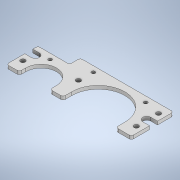
# Autodesk Inventor part: Bottle clamping plate 1
Saved by Autodesk Inventor 2021 (Build 250183000, 183)
## iProperties
Created: 2020-07-28
Part Number: Bottle clamping plate 1
Material: Generic
Document SubType Name: Modeling
Designer: jgray
Density: 1 g/cm^3
Appearance: Default
Author: jgray
Autodesk Inventor part; units mm, degrees
ref_plane "YZ Plane" through (0, 0, 0) normal (1, 0, 0) x (0, 1, 0)
ref_plane "XZ Plane" through (0, 0, 0) normal (0, 1, 0) x (-1, 0, 0)
ref_plane "XY Plane" through (0, 0, 0) normal (0, 0, 1) x (1, 0, 0)
sketch "Sketch1" plane through (0, 0, 0) normal (0, 1, 0) x (-1, 0, 0)
  line L0 (-56.25, 58.25) -> (56.25, 58.25)
  line L1 (56.25, 58.25) -> (56.25, -58.25)
  line L2 (56.25, -58.25) -> (-56.25, -58.25)
  line L3 (-56.25, -58.25) -> (-56.25, 58.25)
  line L4 (-56.25, 58.25) -> (56.25, -58.25) construction
  line L5 (56.25, 58.25) -> (-56.25, -58.25) construction
  point P0 (0, 0)
  dimension "d0" = 112.5
  dimension "d1" = 116.5
  constraints: 12 end point, 2 midpoint, 2 parallel, 1 horizontal, 1 perpendicular
  measures "d0" distance of L1.end L2.end
  measures "d1" distance of L0.end L1.end
extrude "Extrusion1" add sketch "Sketch1" along normal blind 3
sketch "Sketch2" plane through (0, 3, 0) normal (0, 1, 0) x (1, 0, 0)
  circle A0 centre (18.5, 28) radius 23.85
  circle A1 centre (37, -23.25) radius 13.85
  circle A2 centre (-35, -40.25) radius 13.85
  circle A3 centre (-30.9, 25.8) radius 13.85
  circle A4 centre (0, -23.25) radius 13.85
  line L0 (56.25, 58.25) -> (-56.25, 58.25) projected
  line L1 (-56.25, -58.25) -> (56.25, -58.25) projected
  line L2 (0, -105.9299) -> (0, 123.2086) construction
  line L3 (-76.4777, -40.25) -> (-5.35, -40.25) construction
  line L4 (-123.5447, -23.25) -> (82.5572, -23.25) construction
  line L5 (56.25, -58.25) -> (56.25, 58.25) construction
  point P0 (0, 0)
  dimension "d4" = 47.7
  dimension "d5" = 27.7
  dimension "d6" = 27.7
  dimension "d7" = 27.7
  dimension "d8" = 27.7
  dimension "d9" = 116.5
  dimension "d10" = 112.5
  dimension "d13" = 37
  dimension "d14" = 18.5
  dimension "d15" = 30.9
  dimension "d18" = 18
  dimension "d19" = 35
  dimension "d20" = 35
  dimension "d53" = 28
  dimension "d54" = 25.8
  constraints: 6 end point, 5 centre point, 5 point on line, 1 horizontal, 1 perpendicular, 1 vertical
  measures "d4" diameter of A0
  measures "d5" diameter of A1
  measures "d6" diameter of A2
  measures "d7" diameter of A3
  measures "d8" diameter of A4
  measures "d9" distance between parallel lines of L0 L1
  measures "d10" distance of L1.start L1.end
  measures "d13" distance of A4.centre A1.centre
  measures "d14" distance from line of A0.centre L2
  measures "d15" distance from line of A3.centre L2
  measures "d18" distance between parallel lines of L1 L3
  measures "d19" distance between parallel lines of L1 L4
  measures "d20" horizontal distance of A2.centre A4.centre
  measures "d53" vertical distance of point (0, 0) A0.centre
  measures "d54" vertical distance of point (0, 0) A3.centre
extrude "Extrusion2" cut sketch "Sketch2" against normal blind 5
sketch "Sketch4" plane through (0, 3, 0) normal (0, 1, 0) x (1, 0, 0)
  line L0 (-56.25, 58.25) -> (-56.25, -58.25)
  line L1 (56.25, -58.25) -> (56.25, 58.25)
  line L2 (18.5, -17.4904) -> (18.5, -40.0394) construction
  line L3 (-51.55, 5.4) -> (-51.55, 71.9941) construction
  line L4 (50.75, 5.4) -> (50.75, 69.4565) construction
  line L5 (-73.722, 50) -> (66.5467, 50) construction
  line L6 (66.5467, 30) -> (-76.0779, 30) construction
  circle A0 centre (18.5, 28) radius 23.85
  circle A1 centre (37, -23.25) radius 13.85
  circle A2 centre (-30.9, 25.8) radius 13.85
  circle A3 centre (0, -23.25) radius 13.85
  circle A4 centre (-35, -40.25) radius 13.85
  line L7 (56.25, 58.25) -> (-56.25, 58.25)
  line L8 (-56.25, 58.25) -> (-56.25, -58.25)
  line L9 (-56.25, -58.25) -> (56.25, -58.25)
  line L10 (56.25, -58.25) -> (56.25, 58.25)
  circle A5 centre (-30.9, 25.8) radius 13.85
  circle A6 centre (18.5, 28) radius 23.85
  circle A7 centre (0, -23.25) radius 13.85
  circle A8 centre (37, -23.25) radius 13.85
  circle A9 centre (-35, -40.25) radius 13.85
  line L11 (-56.25, 58.25) -> (-56.25, -58.25)
  line L12 (-56.25, 58.25) -> (-56.25, -58.25)
  line L13 (56.25, -58.25) -> (56.25, 58.25)
  line L14 (56.25, 58.25) -> (56.25, -58.25)
  line L15 (-56.25, 20) -> (-44.75, 20)
  line L16 (-17.05, 20) -> (-5.35, 20)
  line L17 (42.35, 20) -> (56.25, 20)
  line L18 (-56.25, -40.25) -> (-48.85, -40.25)
  circle A10 centre (-35, -40.25) radius 13.85
  circle A11 centre (37, -23.25) radius 13.85
  line L19 (50.85, -23.25) -> (56.25, -23.25)
  circle A12 centre (0, -23.25) radius 13.85
  line L20 (-13.85, -23.25) -> (-13.85, -38.25)
  line L21 (-15.85, -40.25) -> (-21.15, -40.25)
  line L22 (13.85, -23.25) -> (13.85, -31.25)
  line L23 (15.85, -33.25) -> (21.15, -33.25)
  line L24 (23.15, -31.25) -> (23.15, -23.25)
  arc A13 (13.85, -31.25) -> (15.85, -33.25) centre (15.85, -31.25) ccw
  arc A14 (21.15, -33.25) -> (23.15, -31.25) centre (21.15, -31.25) ccw
  arc A15 (-15.85, -40.25) -> (-13.85, -38.25) centre (-15.85, -38.25) ccw
  line L25 (-44.75, 25.8) -> (-44.75, 20)
  circle A16 centre (-30.9, 25.8) radius 13.85 projected
  line L26 (-17.05, 25.8) -> (-17.05, 20)
  line L27 (-5.35, 28) -> (-5.35, 20)
  circle A17 centre (18.5, 28) radius 23.85 projected
  line L28 (42.35, 28) -> (42.35, 20)
  line L29 (-110.6194, 0) -> (115.0669, 0) construction
  line L30 (0, -77.0518) -> (0, 133.3252) construction
  point P0 (-56.25, 17.5733)
  point P1 (-42.0273, 17.5733)
  point P2 (-19.7727, 17.5733)
  point P3 (-2.96, 17.5733)
  point P4 (39.1015, 15.9629)
  point P5 (56.25, 15.9629)
  point P6 (-13.85, -23.25)
  point P7 (-21.15, -40.25)
  point P8 (0, 0)
  point P9 (0, 0)
  point P10 (18.5, -13.25)
  point P11 (18.5, -23.25)
  point P12 (-51.55, 30)
  point P13 (50.75, 50)
  point P14 (50.75, 30)
  point P15 (-13.85, -40.25)
  point P16 (13.85, -33.25)
  point P17 (-56.25, 17.5)
  point P18 (-41.9875, 17.5)
  point P19 (-19.8125, 17.5)
  point P20 (-2.9143, 17.5)
  point P21 (39.1112, 16)
  point P22 (56.25, 16)
  point P23 (-21.15, -40.25)
  point P24 (56.25, 20)
  point P25 (-56.25, 20)
  point P26 (56.25, 0)
  point P27 (-56.25, 0)
  point P28 (-11.2, 39.75)
  dimension "d65" = 27.7
  dimension "d55" = 4.7
  dimension "d56" = 5.5
  dimension "d57" = 13.25
  dimension "d58" = 30
  dimension "d59" = 50
  dimension "d60" = 5.4
  dimension "d61" = 5.4
  dimension "d62" = 18.5
  dimension "d63" = 10
  dimension "d64" = 2
  dimension "d66" = 47.7
  dimension "d67" = 2
  dimension "d68" = 27.7
  dimension "d69" = 23.25
  dimension "d70" = 37
  dimension "d73" = 20
  dimension "d88" = 20
  dimension "d89" = 28
  dimension "d98" = 18.5
  dimension "d99" = 45.05
  constraints: 62 end point, 24 point on line, 13 vertical, 10 centre point, 9 perpendicular, 8 point on circle, 8 tangent, 6 coincident, 6 horizontal alignment, 3 horizontal, 2 collinear, 2 line through centre, 2 midpoint, 1 equal radius, 1 parallel, 20 other
  measures "d55" distance from line of L0 L3.start
  measures "d56" distance from line of L1 L4.start
  measures "d57" vertical distance of point (0, 0) point (18.5, -13.25)
  measures "d58" distance from line of point (0, 0) L6
  measures "d59" distance from line of point (0, 0) L5
  measures "d60" vertical distance of point (0, 0) L4.start
  measures "d61" vertical distance of point (0, 0) L3.start
  measures "d62" distance from line of point (0, 0) L2
  measures "d63" distance of L22.start point (13.85, -33.25)
  measures "d64" radius of A13
  measures "d66" diameter of A0
  measures "d67" radius of A15
  measures "d68" diameter of A1
  measures "d69" vertical distance of point (0, 0) A1.centre
  measures "d70" horizontal distance of A1.centre point (0, 0)
  measures "d73" distance from line of point (0, 0) L17
  measures "d88" distance from line of L15.start L29
  measures "d89" distance from line of point (18.5, 28) L29
  measures "d98" distance from line of L7 point (-11.2, 39.75)
  measures "d99" distance from line of L0 point (-11.2, 39.75)
hole "Hole1" at (-51.55, 3, -30) at (50.75, 3, -50) at (50.75, 3, -30) at (-11.2, 3, -39.75) direction (0, -1, 0) diameter 4.2 end through all
extrude "Extrusion3" cut sketch "Sketch4" against normal blind 10 contours L15 L25 A2 L26 L16 L27 A0 L28 L17 L1 L19 A1 L24 A14 L23 A13 L22 A3 L20 A15 L21 A4 L18 L0 | L18 A4 L21 A15 L20 A3 L22 A13 L23 A14 L24 A1 L19 L1 L9 L0
fillet "Fillet1" radius 2 6 edges at (-56.25, 1.5, -20) (-44.75, 1.5, -20) (-17.05, 1.5, -20) (-5.35, 1.5, -20) (42.35, 1.5, -20) (56.25, 1.5, -20)
sketch "Sketch5" plane through (0, 3, 0) normal (0, 1, 0) x (1, 0, 0)
  line L0 (56.25, 58.25) -> (-56.25, 58.25)
  line L1 (56.25, 58.25) -> (-56.25, 58.25)
  line L2 (-46.75, 25.8) -> (-44.75, 25.8)
  arc A0 (-17.05, 25.8) -> (-44.75, 25.8) centre (-30.9, 25.8) ccw
  arc A1 (-17.05, 25.8) -> (-15.05, 27.8) centre (-17.05, 27.8) ccw
  line L3 (-15.05, 27.8) -> (-15.05, 42.25)
  arc A2 (-13.05, 44.25) -> (-15.05, 42.25) centre (-13.05, 42.25) ccw
  line L4 (-13.05, 44.25) -> (-9.35, 44.25)
  arc A3 (-7.35, 42.25) -> (-9.35, 44.25) centre (-9.35, 42.25) ccw
  line L5 (-7.35, 42.25) -> (-7.35, 29.9796)
  arc A4 (-7.35, 29.9796) -> (-5.35, 27.98) centre (-5.35, 29.98) ccw
  arc A5 (42.35, 27.98) -> (-5.35, 27.98) centre (18.5, 28) ccw
  line L6 (42.35, 27.98) -> (44.35, 27.98)
  line L7 (44.35, 27.98) -> (44.35, 58.25)
  line L8 (44.35, 58.25) -> (-46.75, 58.25)
  line L9 (-46.75, 58.25) -> (-46.75, 25.8)
  line L10 (56.25, 58.25) -> (-56.25, 58.25) projected
  point P0 (0, 0)
  point P1 (0, 0)
  point P2 (-40.25, 43.25)
  point P3 (-10.75, 52.75)
  point P4 (36.35, 52.75)
  point P5 (54.25, 58.25)
  point P6 (-54.25, 58.25)
  dimension "d75" = 5.5
  dimension "d76" = 5.5
  dimension "d77" = 15
  dimension "d78" = 6.5
  dimension "d79" = 36
  dimension "d80" = 8
  constraints: 20 end point, 12 point on circle, 6 centre point, 1 collinear
  measures "d75" distance from line of L0 point (36.35, 52.75)
  measures "d76" distance from line of L0 point (-10.75, 52.75)
  measures "d77" distance from line of L1 point (-40.25, 43.25)
  measures "d78" distance from line of point (-40.25, 43.25) L9
  measures "d79" distance from line of point (-10.75, 52.75) L9
  measures "d80" distance from line of point (36.35, 52.75) L7
hole "Hole2" at (-40.25, 3, -43.25) at (-10.75, 3, -52.75) at (36.35, 3, -52.75) direction (0, -1, 0) diameter 3.2 end through all
sketch "Sketch6" plane through (0, 3, 0) normal (0, 1, 0) x (1, 0, 0)
  line L0 (-73.7148, 40) -> (84.1674, 40) construction
  line L1 (56.25, 58.25) -> (-56.25, 58.25) construction
  arc A0 (-50.25, 36.4) -> (-50.25, 43.6) centre (-50.25, 40) ccw
  arc A1 (50.25, 43.6) -> (50.25, 36.4) centre (50.25, 40) ccw
  line L2 (-56.25, 58.25) -> (-56.25, 22) construction
  line L3 (56.25, 22) -> (56.25, 58.25) construction
  line L4 (-50.25, 43.6) -> (-56.25, 43.6)
  line L5 (-50.25, 36.4) -> (-56.25, 36.4)
  line L6 (50.25, 43.6) -> (56.25, 43.6)
  line L7 (56.25, 22) -> (56.25, 58.25) projected
  line L8 (50.25, 36.4) -> (56.25, 36.4)
  line L9 (-56.25, 43.6) -> (-56.25, 36.4)
  point P0 (0, 0)
  point P1 (54.25, 58.25)
  point P2 (-54.25, 58.25)
  point P3 (-56.25, 56.25)
  point P4 (56.25, 56.25)
  dimension "d90" = 18.25
  dimension "d91" = 7.2
  dimension "d92" = 7.2
  dimension "d93" = 6
  dimension "d94" = 6
  constraints: 12 end point, 10 point on line, 4 point on circle, 2 centre point, 2 parallel, 2 tangent, 1 collinear, 1 horizontal
  measures "d90" distance between parallel lines of L1 L0
  measures "d91" diameter of A0
  measures "d92" diameter of A1
  measures "d93" distance from line of L2 A0.centre
  measures "d94" distance from line of L3 A1.centre
extrude "Extrusion4" cut sketch "Sketch6" against normal blind 10
sketch "Sketch7" plane through (0, 3, 0) normal (0, 1, 0) x (1, 0, 0)
  line L0 (-56.25, 58.25) -> (-56.25, 43.6) projected
  line L1 (-27.75, 58.25) -> (-56.25, 58.25)
  line L2 (-56.25, 58.25) -> (-56.25, 48.25)
  line L3 (-56.25, 48.25) -> (-27.75, 48.25)
  line L4 (-27.75, 48.25) -> (-27.75, 58.25)
  line L5 (56.25, 58.25) -> (-56.25, 58.25) projected
  point P0 (0, 0)
  point P1 (-56.25, 56.25)
  point P2 (54.25, 58.25)
  point P3 (-54.25, 58.25)
  point P4 (-56.25, 56.25)
  dimension "d100" = 28.5
  dimension "d101" = 10
  constraints: 8 end point, 2 parallel, 1 collinear, 1 horizontal, 1 perpendicular, 1 point on line
  measures "d100" distance between parallel lines of L4 L0
  measures "d101" distance between parallel lines of L1 L3
extrude "Extrusion5" cut sketch "Sketch7" against normal blind 10
sketch "Sketch8" plane through (56.25, 0, -58.25) normal (0, 0, -1) x (-1, 0, 0)
  line L0 (0, 3) -> (84, 3) projected
  line L1 (0, 0) -> (84, 0) projected
  line L2 (84, 3) -> (0, 3)
  line L3 (0, 3) -> (0, 0)
  line L4 (0, 0) -> (84, 0)
  line L5 (84, 0) -> (84, 3)
  point P0 (56.25, 0)
  constraints: 8 end point, 2 parallel, 1 horizontal, 1 perpendicular
extrude "Extrusion6" cut sketch "Sketch8" against normal blind 0.3
fillet "Fillet3" radius 2 4 edges at (-56.25, 1.5, -48.25) (56.25, 1.5, -57.95) (-27.75, 1.5, -57.95) (-27.75, 1.5, -48.25)
equation "\"d76\" = d75"
body "Solid1"
